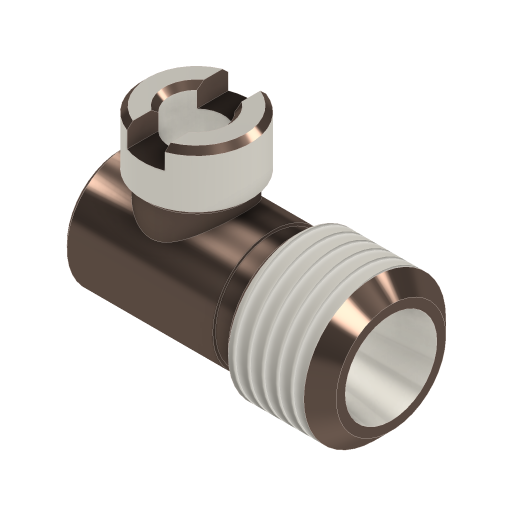
# Autodesk Inventor part: Part020. Hydraulic elbow
Saved by Autodesk Inventor 2023.2 (Build 272271030, 271C)
## iProperties
Created: 2023-09-20
Part Number: Part020. Hydraulic elbow
Material: Steel, Carbon
Document SubType Name: Modeling
Designer: User
Mass: 18.4733 g
Surface Area: 18.6152 cm^2
Volume: 2.35328 cm^3
Density: 7.85 g/cm^3
Appearance: Gunmetal - Antique Polished
Author: User
Autodesk Inventor part; units mm, degrees
ref_plane "YZ Plane" through (0, 0, 0) normal (1, 0, 0) x (0, 1, 0)
ref_plane "XZ Plane" through (0, 0, 0) normal (0, 1, 0) x (-1, 0, 0)
ref_plane "XY Plane" through (0, 0, 0) normal (0, 0, 1) x (1, 0, 0)
sketch "Sketch1" plane through (0, 0, 0) normal (0, 0, 1) x (1, 0, 0)
  line L0 (18, 0) -> (18, 6.5785)
  line L1 (18, 6.5785) -> (9, 6.5785)
  line L2 (9, 6.5785) -> (9, 5.25)
  line L3 (7, 5.5) -> (-7, 5.5)
  line L4 (-7, 5.5) -> (-7, 0)
  line L5 (-7, 0) -> (18, 0)
  line L6 (7, 5.5) -> (7, 5.25)
  line L7 (7, 5.25) -> (9, 5.25)
  point P0 (0, 0)
  dimension "d0" = 25
  dimension "d1" = 18
  dimension "d2" = 11
  dimension "d3" = 10.5
  dimension "d4" = 9
  dimension "d5" = 2
  dimension "d13" = 13.157
  constraints: 16 end point, 7 perpendicular, 1 point on line, 1 vertical
  measures "d0" distance between parallel lines of L0 L4
  measures "d1" distance from line of L0 point (0, 0)
  measures "d2" diameter of L3 L5
  measures "d3" diameter of L7 L5
  measures "d4" distance between parallel lines of L0 L2
  measures "d5" distance of L6.end L2.end
  measures "d13" diameter of L1 L5
revolve "Revolution1" add sketch "Sketch1" angle 360 about axis through (-7, 0, 0) along (1, 0, 0)
chamfer "Chamfer1" distance 1.5 angle 45 1 edges at (18, -6.5785, 0)
chamfer "Chamfer2" distance 0.5 angle 45 1 edges at (9, -6.5785, 0)
thread "Thread1" size "G13.157x1.337" designation "G 1/4" class "A" standard "ISO Pipe Threads" full length
sketch "Sketch2" plane through (0, 0, 0) normal (0, 0, 1) x (1, 0, 0)
  line L0 (0, 12) -> (-5, 12)
  line L1 (-5, 12) -> (-5, 6.5)
  line L2 (-5, 6.5) -> (-4.25, 6.5)
  line L3 (-4.25, 6.5) -> (-4.25, 0)
  line L4 (-4.25, 0) -> (0, 0)
  line L5 (0, 0) -> (0, 12)
  dimension "d16" = 12
  dimension "d17" = 10
  dimension "d18" = 8.5
  dimension "d19" = 5.5
  constraints: 12 end point, 5 perpendicular, 1 horizontal
  measures "d16" distance between parallel lines of L4 L0
  measures "d17" diameter of L1 L5
  measures "d18" diameter of L3 L5
  measures "d19" distance between parallel lines of L2 L0
revolve "Revolution2" add sketch "Sketch2" angle 360 about axis through (0, 0, 0) along (0, 1, 0)
chamfer "Chamfer3" distance 0.5 angle 45 3 edges at (5, 12, 0) (5, 6.5, 0) (-7, -5.5, 0)
sketch "Sketch3" plane through (0, 0, 0) normal (0, 0, 1) x (1, 0, 0)
  line L0 (18, 5.0785) -> (18, -5.0785) projected
  line L1 (18, 0) -> (18, 4.25)
  line L2 (18, 4.25) -> (8.0753, 2.5)
  line L3 (8.0753, 2.5) -> (8.0753, 0)
  line L4 (8.0753, 0) -> (18, 0)
  point P0 (0, 0)
  dimension "d24" = 8.5
  dimension "d25" = 10
  dimension "d26" = 5
  constraints: 8 end point, 1 midpoint, 1 perpendicular, 1 point on line, 1 vertical
  measures "d24" diameter of L1.end L4
  measures "d25" angle of L4 L2
  measures "d26" diameter of L2.end L4
revolve "Revolution3" cut sketch "Sketch3" angle 360 about axis through (8.0753, 0, 0) along (1, 0, 0)
sketch "Sketch4" plane through (18, 0, 0) normal (1, 0, 0) x (0, 0, -1)
  circle A0 centre (0, 0) radius 4.25 projected
  point P0 (0, 0)
  point P1 (0, 0)
  constraints: 1 coincident
hole "Hole1" at (18, 0, 0) direction (-1, 0, 0) diameter 5 depth 20.5 tip angle 118
sketch "Sketch5" plane through (0, 12, 0) normal (0, 1, 0) x (1, 0, 0)
  circle A0 centre (0, 0) radius 4.5 projected
  constraints: 1 coincident
hole "Hole2" at (0, 12, 0) direction (0, -1, 0) diameter 5 depth 14.5 tip angle 118
chamfer "Chamfer4" distance 0.5 angle 45 1 edges at (0, 12, -2.5)
sketch "Sketch6" plane through (0, 0, 0) normal (0, 0, 1) x (1, 0, 0)
  line L0 (-4.5, 12) -> (4.5, 12) projected
  line L1 (-1.75, 12) -> (1.75, 12)
  line L2 (1.75, 12) -> (1.75, 10)
  line L3 (1.75, 10) -> (-1.75, 10)
  line L4 (-1.75, 10) -> (-1.75, 12)
  point P0 (0, 0)
  point P1 (0, 10)
  dimension "d45" = 2
  dimension "d46" = 3.5
  constraints: 8 end point, 2 parallel, 1 horizontal, 1 midpoint, 1 perpendicular, 1 point on line, 1 vertical alignment
  measures "d45" distance between parallel lines of L0 L3
  measures "d46" distance between parallel lines of L2 L4
extrude "Extrusion1" cut sketch "Sketch6" along normal through all both and the other way through all
body "Solid1"
